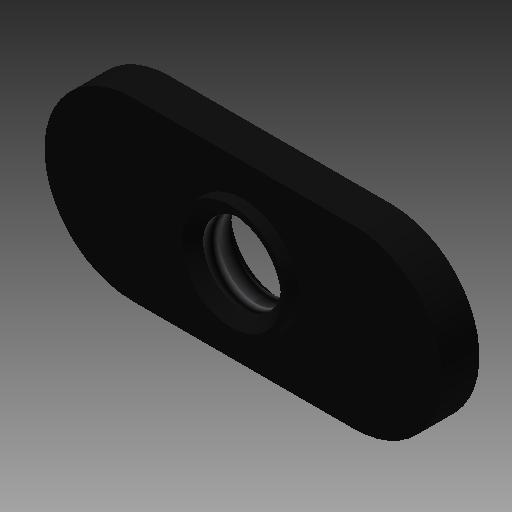
# Autodesk Inventor part: 3382
Saved by Autodesk Inventor 2017 SP1 (Build 210196100, 196)
## iProperties
Category: PARTsolutions
Company: 8020
Created: 2016-04-17
Part Number: 3382
Catalog Web Link: www.cadenas.de
Description: 3275, 3276, 3675, 3382, 3785, 3859, 3686, 3286, 3786, 3836, 3676, 3278, 3778, 3838, 3678-Slide-In Economy T-Nuts
Vendor: 8020
Document SubType Name: Modeling
Designer: psAdmin
Manufacturer: 8020
Mass: 0.578703 g
Surface Area: 6.85304 cm^2
Volume: 0.578703 cm^3
Density: 1 g/cm^3
Material: Generic
Appearance: PSOLRGB-0-0-0
PSOL_IDENT_0: {$CADENAS_DATA\23d-libs\8020\inch\fastening_options\3275.prj},223 {VTYP=3D},{NB=3382},{LINA=3382},{N
PSOL_IDENT_1: N=3275, 3276, 3675, 3382, 3785, 3859, 3686, 3286, 3786, 3836, 3676, 3278, 3778, 3838, 3678},{DATE=22
PSOL_IDENT_2: .08.2012},{GEOMDATE=05.09.2011 00:00:00},{VERSION=},{LINEID=50},{LINESUBID=-1},{WBVAR=}  {NB=3382},{
PSOL_IDENT_3: LINA=3382},{KT=DUMMY},{PN=3382},{NO=4},{NS=Style 1},{A=0.443},{B=1.000},{C=0.094},{D=1/4-20 Centered
PSOL_IDENT_4: },{M=0.2500},{FIN=Black Zinc},{W=.009},{COL=0.00,0.00,0.00,0.00},{X=0.281},{Y=0.030},{Z=0.0000},{R=0
PSOL_IDENT_5: .2215}
NN: 3275, 3276, 3675, 3382, 3785, 3859, 3686, 3286, 3786, 3836, 3676, 3278, 3778, 3838, 3678
NT: Slide-In Economy T-Nuts
NB: 3382
NBSYN: $PN.
LINA: 3382
PN: 3382
NS: Style 1
A: 0.443
B: 1.000
C: 0.094
D: 1/4-20 Centered
FIN: Black Zinc
W: .009
SUPPLIER: 8020
ARTICLENO: 3382
BOMINFO: 3382
CREATOR: CADENAS GmbH
Title: 3382
Author: Cadenas PARTsolutions
Comments: Slide-In Economy T-Nuts
Autodesk Inventor part; units mm, degrees
sketch "Sketch_1" plane through (0, 0, 0) normal (0, 0, 1) x (1, 0, 0)
  arc A0 (-7.0739, 5.6261) -> (-7.0739, -5.6261) centre (-7.0739, 0) ccw
  line L0 (-7.0739, -5.6261) -> (7.0739, -5.6261)
  arc A1 (7.0739, -5.6261) -> (7.0739, 5.6261) centre (7.0739, 0) ccw
  line L1 (7.0739, 5.6261) -> (-7.0739, 5.6261)
  constraints: 4 end point, 4 point on circle, 2 centre point
extrude "Extrusion1" add sketch "Sketch_1" along normal mid plane 2.3876
sketch "Sketch_3" plane through (0, 0, 0) normal (0, 0, 1) x (1, 0, 0)
  circle A0 centre (0, 0) radius 3.5687
  constraints: 1 centre point
extrude "Extrusion2" add sketch "Sketch_3" along normal blind 1.9558
sketch "Sketch_4" plane through (0, 0, 0) normal (1, 0, 0) x (0, 1, 0)
  line L0 (0, -1.1938) -> (0, 1.9558)
  line L1 (0, 1.9558) -> (3.175, 1.9558)
  line L2 (3.175, 1.9558) -> (2.4879, 1.2687)
  line L3 (2.4879, 1.2687) -> (2.4879, -0.5067)
  line L4 (2.4879, -0.5067) -> (3.175, -1.1938)
  line L5 (3.175, -1.1938) -> (0, -1.1938)
  line L6 (0, -1.1938) -> (0, 1.9558)
  constraints: 14 end point
revolve "Revolution1" cut sketch "Sketch_4" angle 360 about axis through (0, 0, -1.1938) along (0, 0, -1)
thread "Thread1" size "1/4-20 UNC" class "2B" standard "ANSI Unified Screw Threads" full length
ref_plane "tnut_XY" through (0, 0, -1.1938) normal (0, 0, 1) x (1, 0, 0)
ref_plane "tnut_YZ" through (0, 0, -1.1938) normal (1, 0, 0) x (0, 1, 0)
ref_plane "tnut_ZX" through (0, 0, -1.1938) normal (0, 1, 0) x (0, 0, 1)
ref_plane "tnut1_XY" through (0, 0, 1.1938) normal (0, 0, 1) x (1, 0, 0)
ref_plane "tnut1_YZ" through (0, 0, 1.1938) normal (1, 0, 0) x (0, 1, 0)
ref_plane "tnut1_ZX" through (0, 0, 1.1938) normal (0, 1, 0) x (0, 0, 1)
body "Solid1"
